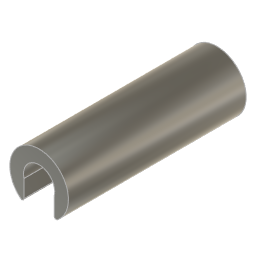
spacer (Autodesk Fusion 360 design; units mm, degrees)
Autodesk Fusion 360 part; units mm, degrees
sketch "Sketch1" plane through (0, 0, 0) normal (0, 1, 0) x (1, 0, 0)
  line L0 (0, -11) -> (0, 10) construction
  line L1 (-3.875, 5.4644) -> (-3.875, 0.9922)
  line L2 (3.875, 0.9922) -> (3.875, 5.4644)
  arc A0 (-4.6875, 5.8547) -> (4.6875, 5.8547) centre (0, 0) ccw
  arc A1 (-3.875, 0.9922) -> (3.875, 0.9922) centre (0, 0) ccw
  arc A2 (-3.875, 5.4644) -> (-4.6875, 5.8547) centre (-4.375, 5.4644) ccw
  arc A3 (4.6875, 5.8547) -> (3.875, 5.4644) centre (4.375, 5.4644) ccw
  dimension "d1" = 8
  dimension "d2" = 15
  dimension "d4" = 0.5
  dimension "d5" = 7.75
  constraint coincident A0.centre A1.centre
  constraint concentric A0 A1
  constraint vertical L0
  constraint parallel L1 L2
  constraint tangent A0 A2
  constraint tangent L1 A2
  constraint tangent L2 A3
  constraint tangent A0 A3
  constraint equal A2 A3
  constraint equal L1 L2
  measures "d1" diameter of A1
  measures "d2" diameter of A0
  measures "d4" radius of A2
  measures "d5" distance of L1 L2
extrude "Extrude1" add sketch "Sketch1" along normal blind 45.5
